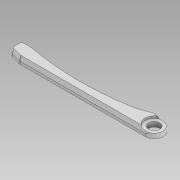
# Autodesk Inventor part: PocketPointBar1
Saved by Autodesk Inventor 2021 (Build 250183000, 183)
## iProperties
Created: 2021-02-18
Part Number: PocketPointBar1
Material: 一般
Document SubType Name: Modeling
Designer: kumagai
Density: 1 g/cm^3
Appearance: 既定
Author: kumagai
Autodesk Inventor part; units mm, degrees
ref_plane "YZ Plane" through (0, 0, 0) normal (1, 0, 0) x (0, 1, 0)
ref_plane "XZ Plane" through (0, 0, 0) normal (0, 1, 0) x (-1, 0, 0)
ref_plane "XY Plane" through (0, 0, 0) normal (0, 0, 1) x (1, 0, 0)
sketch "スケッチ1" plane through (0, 0, 0) normal (0, 1, 0) x (-1, 0, 0)
  line L0 (0, -151.4939) -> (0, 30.1132) projected
  line L1 (-17.6077, 0) -> (76.4346, 0) projected
  arc A0 (0, 4) -> (-0.3541, -3.9843) centre (0, 0) ccw
  line L2 (0, 4) -> (57.4019, 4)
  arc A1 (57.8631, -2.5) -> (12.0944, -2.0253) centre (33.7, -125.55) ccw
  line L3 (63, 2.5) -> (63, -2.5)
  line L4 (-0.3541, -3.9843) -> (4.4833, -4.4142)
  circle A2 centre (0, 0) radius 2.55
  line L5 (63, 2.5) -> (57.4019, 4)
  line L6 (63, -2.5) -> (57.8631, -2.5)
  line L7 (4.4833, -4.4142) -> (10.1243, -2.3699)
  line L8 (10.1243, -2.3699) -> (12.0944, -2.0253)
  dimension "d1" = 8
  dimension "d2" = 129.55
  dimension "d5" = 5.1
  dimension "d12" = 2.5
  dimension "d13" = 2.5
  dimension "d14" = 15
  dimension "d16" = 63
  dimension "d17" = 29.3
  dimension "d23" = 25
  dimension "d24" = 2
  dimension "d25" = 10
  dimension "d26" = 6
  dimension "d28" = 125.4
  constraints: 14 end point, 4 point on circle, 3 centre point, 3 tangent, 2 coincident, 2 horizontal, 1 point on line, 1 vertical
  measures "d1" diameter of A0
  measures "d2" distance from line of A1.centre L2
  measures "d5" diameter of A2
  measures "d12" distance between parallel lines of L6 L1
  measures "d13" distance from line of L1 L3.start
  measures "d14" angle of L2 L5
  measures "d16" distance between parallel lines of L3 L0
  measures "d17" distance from line of A1.centre L3
  measures "d23" angle of L4 L7
  measures "d24" distance of L7.end L8.end
  measures "d25" angle of L7 L8
  measures "d26" distance of L4.end L7.end
  measures "d28" radius of A1
extrude "押し出し1" add sketch "スケッチ1" along normal blind 3.2 contours L4 A0 L1 A2 L0 | L0 A2 L1 L3 L6 A1 L8 L7 L4 | L1 A0 L0 A2 | A2 L0 L2 L5 L3 L1
fillet "フィレット1" radius 1.5 6 edges at (-63, 1.6, 2.5) (-57.4019, 1.6, 4) (-63, 1.6, -2.5) (-57.8631, 1.6, -2.5) (-4.4833, 1.6, -4.4142) (-10.1243, 1.6, -2.3699)
sketch "スケッチ2" plane through (0, 3.2, 0) normal (0, 1, 0) x (1, 0, 0)
  circle A0 centre (0, 0) radius 4.25
  dimension "d9" = 8.5
  constraints: 1 centre point, 1 coincident
  measures "d9" diameter of A0
extrude "押し出し2" cut sketch "スケッチ2" against normal blind 1
chamfer "面取り1" distance 0.5 distance2 2 10 edges at (-29.3203, 3.2, 4) (-57.4002, 3.2, 3.9872) (-59.7405, 3.2, 3.3734) (-62.69, 3.2, 2.2622) (-63, 3.2, 0.1745) (-62.5607, 3.2, -2.0607) (-59.7543, 3.2, -2.5) (-57.8643, 3.2, -2.493) (-34.9283, 3.2, -0.156) (-2.6143, 3.2, -4.2481) measured on face at (-59.7543, 3.2, -2) measured on face at (-57.9124, 3.2, -1.9954) measured on face at (-59.611, 3.2, 2.8904) measured on face at (-34.9332, 3.2, 0.344) measured on face at (-57.335, 3.2, 3.4914) measured on face at (-2.6585, 3.2, -3.7501) measured on face at (-62.2071, 3.2, -1.7071) measured on face at (-29.3203, 3.2, 3.5) measured on face at (-62.2934, 3.2, 1.9578) measured on face at (-62.5, 3.2, 0.1745)
